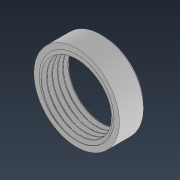
# Autodesk Inventor part: topPiece
Saved by Autodesk Inventor 2022 (Build 260153000, 153)
## iProperties
Created: 2022-07-02
Part Number: topPiece
Material: Generic
Document SubType Name: Modeling
Designer: User
Density: 1 g/cm^3
Appearance: Default
Author: User
## iProperties of the stored document topPiece_3DPrint.ipt
Created: 2022-07-04
Part Number: topPiece_3DPrint
Material: Generic
Document SubType Name: Modeling
Designer: User
Density: 1 g/cm^3
Appearance: Default
Author: User
Autodesk Inventor part; units mm, degrees
ref_plane "YZ Plane" through (0, 0, 0) normal (1, 0, 0) x (0, 1, 0)
ref_plane "XZ Plane" through (0, 0, 0) normal (0, 1, 0) x (-1, 0, 0)
ref_plane "XY Plane" through (0, 0, 0) normal (0, 0, 1) x (1, 0, 0)
sketch "Sketch1" plane through (0, 0, 0) normal (0, 0, 1) x (1, 0, 0)
  circle A0 centre (0, 0) radius 14
  circle A1 centre (0, 0) radius 16
  dimension "d0" = 28
  dimension "d1" = 32
  constraints: 2 centre point, 2 coincident
  measures "d0" diameter of A0
  measures "d1" diameter of A1
extrude "Extrusion1" add sketch "Sketch1" along normal blind 10
thread "M28x2" size "M28x2" class "6H" standard "ANSI Metric M Profile" full length
chamfer "Chamfer1" [suppressed]
sketch "Sketch7" plane through (0, 0, 10) normal (-1, 0, 0) x (0, 1, 0)
  line L0 (14, 0) -> (14, 10)
  line L1 (14, 10) -> (12.5171, 10)
  line L2 (12.5171, 10) -> (12.5171, 0)
  line L3 (12.5171, 0) -> (14, 0)
  line L4 (0, -4.6171) -> (0, 12.4362) projected
  constraints: 8 end point
revolve "Revolution3" add sketch "Sketch7" angle 360 about axis through (0, 0, 10) along (0, 0, -1) separate body
sketch "Sketch6" plane through (0, 14, 10) normal (1, 0, 0) x (0, 0, -1)
  line L0 (-1.1668, -0.1013) -> (-1.0001, -0.1013) construction
  line L1 (0.1666, -1.382) -> (-0.0001, -1.7021) construction
  line L2 (-2.0001, -1.7021) -> (-2.1668, -1.382) construction
  line L3 (-0.8334, -0.1013) -> (-1.0001, 0.2189) construction
  line L4 (-1.0001, 0.2189) -> (-1.1668, -0.1013) construction
  line L5 (-2.0001, -1.7021) -> (-1.8334, -1.382) construction
  line L6 (-0.8334, -0.1013) -> (-0.1668, -1.382)
  line L7 (-2.1668, -1.382) -> (-1.8334, -1.382) construction
  arc A0 (-2.1668, -1.382) -> (-2.0001, -1.4831) centre (-2.0001, -1.2952) ccw construction
  line L8 (0.1666, -1.382) -> (-0.1668, -1.382) construction
  line L9 (-2.0001, -1.7021) -> (-2.0001, -1.382) construction
  line L10 (-0.0001, -1.7021) -> (-0.0001, -1.382) construction
  line L11 (-1.0001, 0.2189) -> (-1.0001, -0.0002) construction
  line L12 (-2.0001, -1.4831) -> (-0.0001, -1.4831)
  arc A1 (-2.0001, -1.4831) -> (-1.8334, -1.382) centre (-2.0001, -1.2952) ccw
  line L13 (-0.1668, -1.382) -> (-0.0001, -1.7021) construction
  line L14 (-1.8334, -1.382) -> (-1.1668, -0.1013)
  line L15 (-0.0001, -0.0002) -> (-0.0001, 0.0177)
  line L16 (-0.0001, 0.0177) -> (-0.0001, -0.0002)
  line L17 (-0.0001, -0.0002) -> (0.0334, -0.0002)
  arc A2 (-0.1668, -1.382) -> (-0.0001, -1.4831) centre (-0.0001, -1.2952) ccw
  arc A3 (-0.0001, -1.4831) -> (0.1666, -1.382) centre (-0.0001, -1.2952) ccw construction
  arc A4 (-1.0001, -0.0002) -> (-1.1668, -0.1013) centre (-1.0001, -0.1881) ccw
  arc A5 (-0.8334, -0.1013) -> (-1.0001, -0.0002) centre (-1.0001, -0.1881) ccw
  line L18 (-1.0001, -0.0002) -> (-1.0001, -0.1013) construction
  line L19 (-1.0001, -0.1013) -> (-0.8334, -0.1013) construction
  dimension "d47" = 55
  dimension "d48" = 0.3202
  dimension "d49" = 0.3202
  dimension "Sketch6_ThreadOffset" = 0
  dimension "Sketch6_MajorRadius" = 1.4829
  dimension "d52" = 2
  dimension "Sketch6_MinorRadius" = 0
  constraints: 40 end point, 12 point on circle, 10 parallel, 8 tangent, 6 centre point, 6 collinear, 2 midpoint, 2 point on line, 1 horizontal, 1 perpendicular, 3 other
  measures "d47" angle of L6 L14
  measures "d48" distance of L3.end L0.end
  measures "d49" distance of L1.end L10.end
  measures "Sketch6_ThreadOffset" distance between parallel lines of L15 L10
  measures "Sketch6_MajorRadius" distance from line of L12 L15.start
  measures "d52" distance from line of L1.end L9
  measures "Sketch6_MinorRadius" distance edge to line of A5 L17
coil "Coil3" sketch "Sketch6" operation cut axis through (0, 0, 10) along (0, 0, -1) pitch 2.002 turns 6.993007 hand right bodies 2
chamfer "Chamfer2" distance 1 angle 45 1 edges at (-16, 0, 0)
equation "\"d47\" = d54"
equation "\"d48\" = 0.160083 * Sketch6_Pitch"
equation "\"d49\" = 0.160083 * Sketch6_Pitch"
equation "\"d52\" = Sketch6_Pitch"
equation "\"d13\" = 55deg"
equation "\"Sketch2_Pitch\" = 1.5"
equation "\"d33\" = 55deg"
equation "\"Sketch4_Pitch\" = 2"
equation "\"d54\" = 55deg"
equation "\"Sketch6_Pitch\" = 2"
body "Solid1"
body "Solid4"
